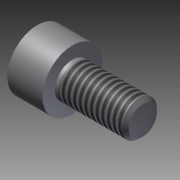
# Autodesk Inventor part: CBM5-10
Saved by Autodesk Inventor 2013 (Build 170138000, 138)
## iProperties
Category: PARTsolutions
Company: MISUMI
Created: 2013-06-20
Part Number: CBM5-10
Catalog Web Link: www.cadenas.de
Description: CBM-Hexagon Socket Head Cap Screws - Bright Chromate
Vendor: MISUMI
Document SubType Name: Modeling
Designer: PARTuser1
Manufacturer: MISUMI
Density: 1 g/cm^3
Material: Generic
PSOL_IDENT_0: {\\10.0.0.242\data_v8\23d-libs\misumi\metric\27_screws_nuts\cbm.prj},154 {VTYP=3D},{NB=CBM5-10},{LIN
PSOL_IDENT_1: A=CBM5-10},{NN=CBM},{DATE=15.01.2013 05:07:40},{GEOMDATE=10.06.2010 00:00:00},{VERSION=},{LINEID=40}
PSOL_IDENT_2: ,{LINESUBID=-1},{WBVAR=L}  {NB=CBM5-10},{LINA=CBM5-10},{KT=DUMMY},{PN=CBM5-10},{MAT=4137 Steel},{ST=
PSOL_IDENT_3: Bright Chromate},{M=5},{L=10},{LL=Full Thread},{L1=22},{TYPE=CBM},{M1=5},{L0=8,10,12,14,15,18,20,22,
PSOL_IDENT_4: 25,30,35,40,45,50},{NDM=5},{KDM=4.017064},{MP=5x0.8},{P=0.8},{A=8.5},{E=5.0},{B=4.0}
SUPPLIER: MISUMI
ARTICLENO: CBM5-10
BOMINFO: CBM5-10
CREATOR: CADENAS GmbH
Title: CBM5-10
Author: Cadenas PARTsolutions
Comments: Hexagon Socket Head Cap Screws - Bright Chromate
Autodesk Inventor part; units mm, degrees
sketch "Sketch_1" plane through (0, 0, 0) normal (0, 0, 1) x (1, 0, 0)
  line L0 (10, 0) -> (-5, 0)
  line L1 (-5, 0) -> (-5, 4.25)
  line L2 (-5, 4.25) -> (0, 4.25)
  line L3 (0, 4.25) -> (0, 2.5)
  line L4 (0, 2.5) -> (9.5095, 2.5)
  line L5 (9.5095, 2.5) -> (10, 2.0095)
  line L6 (10, 2.0095) -> (10, 0)
  line L7 (10, 0) -> (-5, 0)
  constraints: 16 end point
revolve "Revolution1" add sketch "Sketch_1" angle 360 about axis through (10, 0, 0) along (1, 0, 0)
thread "Thread1" size "M5x0.8" class "6g" standard "ISO Metric profile" length 9.5 offset 0.5
sketch "Sketch_4" plane through (0, 0, 0) normal (0, 0, 1) x (1, 0, 0)
  line L0 (-1.9641, 0) -> (-5, 0)
  line L1 (-5, 0) -> (-5, 2)
  line L2 (-5, 2) -> (-2.5, 2)
  line L3 (-2.5, 2) -> (-1.9641, 0)
  line L4 (-1.9641, 0) -> (-5, 0)
  constraints: 10 end point
revolve "Revolution2" cut sketch "Sketch_4" angle 360 about axis through (-1.9641, 0, 0) along (1, 0, 0)
sketch "Sketch_3" plane through (-5, 0, 0) normal (1, 0, 0) x (0, 0, -1)
  line L0 (-2, 1.1547) -> (-2, -1.1547)
  line L1 (-2, -1.1547) -> (0, -2.3094)
  line L2 (0, -2.3094) -> (2, -1.1547)
  line L3 (2, -1.1547) -> (2, 1.1547)
  line L4 (2, 1.1547) -> (0, 2.3094)
  line L5 (0, 2.3094) -> (-2, 1.1547)
  constraints: 12 end point
extrude "Extrusion1" cut sketch "Sketch_3" along normal blind 2.5
ref_plane "bolt_XY" through (0, 0, 0) normal (1, 0, 0) x (0, 0, -1)
ref_plane "bolt_YZ" through (0, 0, 0) normal (0, 0, -1) x (0, 1, 0)
ref_plane "bolt_ZX" through (0, 0, 0) normal (0, 1, 0) x (1, 0, 0)
ref_plane "nut_XY" through (10, 0, 0) normal (1, 0, 0) x (0, 0, -1)
ref_plane "nut_YZ" through (10, 0, 0) normal (0, 0, -1) x (0, 1, 0)
ref_plane "nut_ZX" through (10, 0, 0) normal (0, 1, 0) x (1, 0, 0)
body "Solid1"
